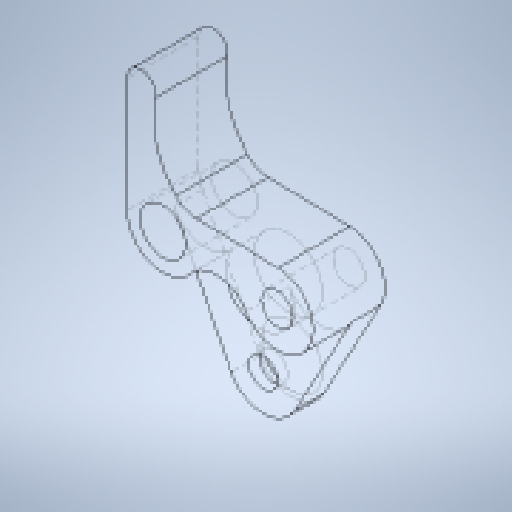
# Autodesk Inventor part: Lever
Saved by Autodesk Inventor 2023.2 (Build 272271000, 271)
## iProperties
Created: 2024-01-16
Part Number: Lever
Material: Aluminum 6061
Document SubType Name: Modeling
Designer: Nathan Cai
Mass: 3.70951 g
Surface Area: 13.9952 cm^2
Volume: 1.37389 cm^3
Density: 2.7 g/cm^3
Appearance: Aluminum - Flat
Lever_Offset: 0.500 in
Lever_Angle: 95.00 deg
Author: Nathan Cai
Autodesk Inventor part; units mm, degrees
ref_plane "YZ Plane" through (0, 0, 0) normal (1, 0, 0) x (0, 1, 0)
ref_plane "XZ Plane" through (0, 0, 0) normal (0, 1, 0) x (-1, 0, 0)
ref_plane "XY Plane" through (0, 0, 0) normal (0, 0, 1) x (1, 0, 0)
sketch "Sketch4" plane through (0, 0, 0) normal (0, 0, 1) x (1, 0, 0)
  circle A0 centre (0, 0) radius 2.5083
  circle A1 centre (0, 0) radius 3.9688
  line L0 (-3.9688, 0) -> (-3.9688, 12.7)
  arc A2 (-0.8259, 12.3821) -> (-3.9688, 12.7) centre (-2.3812, 12.7) ccw
  arc A3 (-0.8259, 12.3821) -> (2.5018, 3.0809) centre (8.5062, 10.475) ccw
  circle A4 centre (0, 0) radius 4.7625 construction
  circle A5 centre (12.6517, -1.1069) radius 6.35 construction
  circle A6 centre (12.6517, -1.1069) radius 3.9688
  circle A7 centre (12.6517, -1.1069) radius 1.7526
  line L1 (2.5018, 3.0809) -> (12.7369, 2.861)
  circle A8 centre (6.35, -12.7) radius 3.9688
  circle A9 centre (6.35, -12.7) radius 1.5875
  line L2 (2.8002, -14.4749) -> (-3.5498, -1.7749)
  circle A10 centre (5.9396, -4.9677) radius 3.7745
  line L3 (16.1386, -3.0023) -> (9.8369, -14.5954)
  line L4 (0, 0) -> (12.6517, -1.1069) construction
  line L5 (12.6517, -1.1069) -> (12.9976, 2.8468) construction
  line L6 (0, 4.7625) -> (0, 0) construction
  point P0 (3.9688, 0)
  point P1 (9.8232, -3.8909)
  point P2 (2.0561, -3.3946)
  point P3 (3.0443, -2.5462)
  point P4 (9.2114, -3.0857)
  dimension "d54" = 9.525
  dimension "d44" = 5.0165
  dimension "d45" = 7.9375
  dimension "d51" = 12.7
  dimension "d52" = 3.175
  dimension "d53" = 9.525
  dimension "d56" = 12.7
  dimension "d57" = 7.9375
  dimension "d58" = 3.5052
  dimension "d61" = 7.9375
  dimension "d62" = 3.175
  dimension "d63" = 12.7
  dimension "d64" = 6.35
  dimension "Lever_Offset" = 12.7
  dimension "Lever_Angle" = 95
  constraints: 15 point on circle, 14 end point, 12 tangent, 10 centre point, 6 coincident, 2 vertical, 1 perpendicular, 1 vertical alignment, 2 other
  measures "d44" diameter of A0
  measures "d45" diameter of A1
  measures "d51" distance of L0.start L0.end
  measures "d52" diameter of A2
  measures "d53" radius of A3
  measures "d56" diameter of A5
  measures "d57" diameter of A6
  measures "d58" diameter of A7
  measures "d61" diameter of A8
  measures "d62" diameter of A9
  measures "d63" vertical distance of A1.centre A8.centre
  measures "d64" horizontal distance of A0.centre A8.centre
  measures "Lever_Offset" distance from line of point (0, 0) L5
  measures "Lever_Angle" angle of L6 L4
extrude "Extrusion3" add sketch "Sketch4" along normal blind 7.9375 contours A1 | A1 L1 A6 A10 | A1 L0 A2 A3 | A10 A8 L2 A1 | A6 | A6 L3 A8 A10 | A8
fillet "Fillet5" radius 3.175 1 edges at (2.5018, 3.0809, 3.9688)
sketch "Sketch5" plane through (0, 0, 7.9375) normal (0, 0, 1) x (1, 0, 0)
  circle A0 centre (5.9396, -4.9677) radius 3.7745 projected
  circle A1 centre (0, 0) radius 2.5083 projected
  circle A2 centre (12.6517, -1.1069) radius 1.7526 projected
  circle A3 centre (6.35, -12.7) radius 1.5875 projected
  arc A4 (16.1386, -3.0023) -> (12.7369, 2.861) centre (12.6517, -1.1069) ccw projected
  line L0 (12.7369, 2.861) -> (3.7163, 3.0548) projected
  arc A5 (1.4237, 4.1061) -> (3.7163, 3.0548) centre (3.7845, 6.2291) ccw projected
  arc A6 (-0.8259, 12.3821) -> (1.4237, 4.1061) centre (8.5062, 10.475) ccw projected
  arc A7 (-0.8259, 12.3821) -> (-3.9687, 12.7) centre (-2.3812, 12.7) ccw projected
  line L1 (-3.9687, 12.7) -> (-3.9687, 0) projected
  arc A8 (-3.9687, 0) -> (-3.5498, -1.7749) centre (0, 0) ccw projected
  line L2 (-3.5498, -1.7749) -> (2.8002, -14.4749) projected
  arc A9 (2.8002, -14.4749) -> (9.8369, -14.5954) centre (6.35, -12.7) ccw projected
  line L3 (9.8369, -14.5954) -> (16.1386, -3.0023) projected
  circle A10 centre (6.35, -12.7) radius 3.9688
  circle A11 centre (5.9396, -4.9677) radius 3.7745 projected
  circle A12 centre (0, 0) radius 3.9688
  circle A13 centre (12.6517, -1.1069) radius 3.9687
  point P0 (3.0443, -2.5462)
  point P1 (-3.5498, -1.7749)
  point P2 (9.2114, -3.0857)
  constraints: 3 centre point, 3 coincident, 3 tangent
extrude "Extrusion4" cut sketch "Sketch5" against normal blind 4.7625 contours A0 A13 L3 A10 | A10 L2 A12 A0 | A10 A9
chamfer "Chamfer2" distance 1.778 angle 49 1 edges at (4.7625, -12.7, 0) measured on face at (4.2625, -12.7, 0)
body "Solid2"
